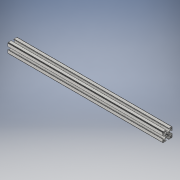
# Autodesk Inventor part: 30x30_extrude_horizontal_481mm
Saved by Autodesk Inventor 2016 (Build 200138000, 138)
## iProperties
Created: 2016-10-05
Part Number: 30x30_extrude_horizontal_481mm
Material: Generic
Document SubType Name: Modeling
Designer: gmmar
Density: 1 g/cm^3
Appearance: Default
Author: gmmar
Autodesk Inventor part; units mm, degrees
ref_plane "YZ Plane" through (0, 0, 0) normal (1, 0, 0) x (0, 1, 0)
ref_plane "XZ Plane" through (0, 0, 0) normal (0, 1, 0) x (-1, 0, 0)
ref_plane "XY Plane" through (0, 0, 0) normal (0, 0, 1) x (1, 0, 0)
sketch "Sketch1" plane through (0, 0, 0) normal (1, 0, 0) x (0, 1, 0)
  line L0 (12.7969, -8.25) -> (12.7969, -4)
  line L1 (-12.8031, 4) -> (-12.8031, 8.25)
  line L2 (-13.849, -12.8949) -> (-13.85, -12.85)
  line L3 (9.701, -12.8949) -> (9.7, -12.85)
  line L4 (-9.7, -10.7) -> (-9.701, -10.6551)
  line L5 (13.85, -10.7) -> (13.849, -10.6551)
  line L6 (9.701, 10.6551) -> (9.7, 10.7)
  line L7 (-13.849, 10.6551) -> (-13.85, 10.7)
  line L8 (13.85, 12.85) -> (13.849, 12.8949)
  line L9 (-9.7, 12.85) -> (-9.701, 12.8949)
  line L10 (-14.998, -13.0897) -> (-15, -13)
  line L11 (15, 13) -> (14.998, 13.0897)
  line L12 (9.704, -12.9396) -> (9.701, -12.8949)
  line L13 (-9.701, -10.6551) -> (-9.704, -10.6104)
  line L14 (9.704, 10.6104) -> (9.701, 10.6551)
  line L15 (-9.701, 12.8949) -> (-9.704, 12.9396)
  line L16 (-14.9919, -13.1793) -> (-14.998, -13.0897)
  line L17 (14.998, 13.0897) -> (14.9919, 13.1793)
  line L18 (-13.846, -12.9396) -> (-13.849, -12.8949)
  line L19 (13.849, -10.6551) -> (13.846, -10.6104)
  line L20 (-13.846, 10.6104) -> (-13.849, 10.6551)
  line L21 (13.849, 12.8949) -> (13.846, 12.9396)
  line L22 (13.846, -10.6104) -> (13.8409, -10.5658)
  line L23 (-13.8409, 10.5658) -> (-13.846, 10.6104)
  line L24 (-13.8409, -12.9842) -> (-13.846, -12.9396)
  line L25 (13.846, 12.9396) -> (13.8409, 12.9842)
  line L26 (-14.9819, -13.2685) -> (-14.9919, -13.1793)
  line L27 (14.9919, 13.1793) -> (14.9819, 13.2685)
  line L28 (-9.704, -10.6104) -> (-9.7091, -10.5658)
  line L29 (9.7091, 10.5658) -> (9.704, 10.6104)
  line L30 (9.7091, -12.9842) -> (9.704, -12.9396)
  line L31 (-9.704, 12.9396) -> (-9.7091, 12.9842)
  line L32 (-13.8339, -13.0286) -> (-13.8409, -12.9842)
  line L33 (9.7161, -13.0286) -> (9.7091, -12.9842)
  line L34 (13.8409, 12.9842) -> (13.8339, 13.0286)
  line L35 (-9.7091, 12.9842) -> (-9.7161, 13.0286)
  line L36 (-14.9679, -13.3571) -> (-14.9819, -13.2685)
  line L37 (14.9819, 13.2685) -> (14.9679, 13.3571)
  line L38 (-9.7091, -10.5658) -> (-9.7161, -10.5214)
  line L39 (13.8409, -10.5658) -> (13.8339, -10.5214)
  line L40 (9.7161, 10.5214) -> (9.7091, 10.5658)
  line L41 (-13.8339, 10.5214) -> (-13.8409, 10.5658)
  line L42 (-14.9499, -13.445) -> (-14.9679, -13.3571)
  line L43 (14.9679, 13.3571) -> (14.9499, 13.445)
  line L44 (-13.8249, -13.0725) -> (-13.8339, -13.0286)
  line L45 (9.7251, -13.0725) -> (9.7161, -13.0286)
  line L46 (-9.7161, -10.5214) -> (-9.7251, -10.4775)
  line L47 (13.8339, -10.5214) -> (13.8249, -10.4775)
  line L48 (9.7251, 10.4775) -> (9.7161, 10.5214)
  line L49 (-13.8249, 10.4775) -> (-13.8339, 10.5214)
  line L50 (13.8339, 13.0286) -> (13.8249, 13.0725)
  line L51 (-9.7161, 13.0286) -> (-9.7251, 13.0725)
  line L52 (-14.9279, -13.5321) -> (-14.9499, -13.445)
  line L53 (-9.7251, -10.4775) -> (-9.736, -10.434)
  line L54 (13.8249, -10.4775) -> (13.814, -10.434)
  line L55 (9.736, 10.434) -> (9.7251, 10.4775)
  line L56 (-13.814, 10.434) -> (-13.8249, 10.4775)
  line L57 (14.9499, 13.445) -> (14.9279, 13.5321)
  line L58 (-13.814, -13.116) -> (-13.8249, -13.0725)
  line L59 (9.736, -13.116) -> (9.7251, -13.0725)
  line L60 (13.8249, 13.0725) -> (13.814, 13.116)
  line L61 (-9.7251, 13.0725) -> (-9.736, 13.116)
  line L62 (-13.8011, -13.159) -> (-13.814, -13.116)
  line L63 (9.7489, -13.159) -> (9.736, -13.116)
  line L64 (13.814, 13.116) -> (13.8011, 13.159)
  line L65 (-9.736, 13.116) -> (-9.7489, 13.159)
  line L66 (-9.736, -10.434) -> (-9.7489, -10.391)
  line L67 (13.814, -10.434) -> (13.8011, -10.391)
  line L68 (9.7489, 10.391) -> (9.736, 10.434)
  line L69 (-13.8011, 10.391) -> (-13.814, 10.434)
  line L70 (-14.9021, -13.618) -> (-14.9279, -13.5321)
  line L71 (14.9279, 13.5321) -> (14.9021, 13.618)
  line L72 (-14.8725, -13.7027) -> (-14.9021, -13.618)
  line L73 (14.9021, 13.618) -> (14.8725, 13.7027)
  line L74 (-13.7862, -13.2014) -> (-13.8011, -13.159)
  line L75 (9.7638, -13.2014) -> (9.7489, -13.159)
  line L76 (-9.7489, -10.391) -> (-9.7638, -10.3486)
  line L77 (13.8011, -10.391) -> (13.7862, -10.3486)
  line L78 (9.7638, 10.3486) -> (9.7489, 10.391)
  line L79 (-13.7862, 10.3486) -> (-13.8011, 10.391)
  line L80 (13.8011, 13.159) -> (13.7862, 13.2014)
  line L81 (-9.7489, 13.159) -> (-9.7638, 13.2014)
  line L82 (-14.8391, -13.7861) -> (-14.8725, -13.7027)
  line L83 (14.8725, 13.7027) -> (14.8391, 13.7861)
  line L84 (9.7805, -13.243) -> (9.7638, -13.2014)
  line L85 (-9.7638, -10.3486) -> (-9.7805, -10.307)
  line L86 (9.7805, 10.307) -> (9.7638, 10.3486)
  line L87 (-9.7638, 13.2014) -> (-9.7805, 13.243)
  line L88 (-13.7695, -13.243) -> (-13.7862, -13.2014)
  line L89 (13.7862, -10.3486) -> (13.7695, -10.307)
  line L90 (-13.7695, 10.307) -> (-13.7862, 10.3486)
  line L91 (13.7862, 13.2014) -> (13.7695, 13.243)
  line L92 (-13.751, -13.2839) -> (-13.7695, -13.243)
  line L93 (13.7695, -10.307) -> (13.751, -10.2661)
  line L94 (-13.751, 10.2661) -> (-13.7695, 10.307)
  line L95 (13.7695, 13.243) -> (13.751, 13.2839)
  line L96 (9.799, -13.2839) -> (9.7805, -13.243)
  line L97 (-9.7805, -10.307) -> (-9.799, -10.2661)
  line L98 (9.799, 10.2661) -> (9.7805, 10.307)
  line L99 (-9.7805, 13.243) -> (-9.799, 13.2839)
  line L100 (-14.8019, -13.8678) -> (-14.8391, -13.7861)
  line L101 (14.8391, 13.7861) -> (14.8019, 13.8678)
  line L102 (-13.7306, -13.3239) -> (-13.751, -13.2839)
  line L103 (13.751, -10.2661) -> (13.7306, -10.2261)
  line L104 (-13.7306, 10.2261) -> (-13.751, 10.2661)
  line L105 (13.751, 13.2839) -> (13.7306, 13.3239)
  line L106 (-14.7612, -13.9477) -> (-14.8019, -13.8678)
  line L107 (14.8019, 13.8678) -> (14.7612, 13.9477)
  line L108 (9.8194, -13.3239) -> (9.799, -13.2839)
  line L109 (-9.799, -10.2661) -> (-9.8194, -10.2261)
  line L110 (9.8194, 10.2261) -> (9.799, 10.2661)
  line L111 (-9.799, 13.2839) -> (-9.8194, 13.3239)
  line L112 (-9.8194, -10.2261) -> (-9.8416, -10.1871)
  line L113 (9.8416, 10.1871) -> (9.8194, 10.2261)
  line L114 (9.8416, -13.3629) -> (9.8194, -13.3239)
  line L115 (-9.8194, 13.3239) -> (-9.8416, 13.3629)
  line L116 (-14.7169, -14.0258) -> (-14.7612, -13.9477)
  line L117 (14.7612, 13.9477) -> (14.7169, 14.0258)
  line L118 (13.7306, -10.2261) -> (13.7084, -10.1871)
  line L119 (-13.7084, 10.1871) -> (-13.7306, 10.2261)
  line L120 (-13.7084, -13.3629) -> (-13.7306, -13.3239)
  line L121 (13.7306, 13.3239) -> (13.7084, 13.3629)
  line L122 (6, -0.9196) -> (5.4782, 0)
  line L123 (-5.4782, 0) -> (-6, 0.9196)
  line L124 (-13.6846, -13.4009) -> (-13.7084, -13.3629)
  line L125 (13.7084, 13.3629) -> (13.6846, 13.4009)
  line L126 (13.7084, -10.1871) -> (13.6846, -10.1491)
  line L127 (-13.6846, 10.1491) -> (-13.7084, 10.1871)
  line L128 (-14.6691, -14.1018) -> (-14.7169, -14.0258)
  line L129 (14.7169, 14.0258) -> (14.6691, 14.1018)
  line L130 (9.8654, -13.4009) -> (9.8416, -13.3629)
  line L131 (-9.8416, 13.3629) -> (-9.8654, 13.4009)
  line L132 (-9.8416, -10.1871) -> (-9.8654, -10.1491)
  line L133 (9.8654, 10.1491) -> (9.8416, 10.1871)
  line L134 (-13.659, -13.4378) -> (-13.6846, -13.4009)
  line L135 (9.891, -13.4378) -> (9.8654, -13.4009)
  line L136 (-9.8654, -10.1491) -> (-9.891, -10.1122)
  line L137 (13.6846, -10.1491) -> (13.659, -10.1122)
  line L138 (9.891, 10.1122) -> (9.8654, 10.1491)
  line L139 (-13.659, 10.1122) -> (-13.6846, 10.1491)
  line L140 (13.6846, 13.4009) -> (13.659, 13.4378)
  line L141 (-9.8654, 13.4009) -> (-9.891, 13.4378)
  line L142 (-14.618, -14.1756) -> (-14.6691, -14.1018)
  line L143 (14.6691, 14.1018) -> (14.618, 14.1756)
  line L144 (-4.3624, -3.3495) -> (-4.5314, -3.1172)
  line L145 (4.5284, 3.125) -> (4.3639, 3.3512)
  line L146 (9.9182, -13.4735) -> (9.891, -13.4378)
  line L147 (-9.891, -10.1122) -> (-9.9182, -10.0765)
  line L148 (9.9182, 10.0765) -> (9.891, 10.1122)
  line L149 (-9.891, 13.4378) -> (-9.9182, 13.4735)
  line L150 (-14.5637, -14.247) -> (-14.618, -14.1756)
  line L151 (14.618, 14.1756) -> (14.5637, 14.247)
  line L152 (-13.6318, -13.4735) -> (-13.659, -13.4378)
  line L153 (13.659, -10.1122) -> (13.6318, -10.0765)
  line L154 (-13.6318, 10.0765) -> (-13.659, 10.1122)
  line L155 (13.659, 13.4378) -> (13.6318, 13.4735)
  line L156 (-4.1783, -3.57) -> (-4.3624, -3.3495)
  line L157 (4.3639, 3.3512) -> (4.1798, 3.5718)
  line L158 (-14.5061, -14.3159) -> (-14.5637, -14.247)
  line L159 (13.6318, -10.0765) -> (13.6031, -10.0421)
  line L160 (-13.6031, 10.0421) -> (-13.6318, 10.0765)
  line L161 (14.5637, 14.247) -> (14.5061, 14.3159)
  line L162 (-13.6031, -13.5079) -> (-13.6318, -13.4735)
  line L163 (13.6318, 13.4735) -> (13.6031, 13.5079)
  line L164 (-9.9182, -10.0765) -> (-9.9469, -10.0421)
  line L165 (9.9469, 10.0421) -> (9.9182, 10.0765)
  line L166 (9.9469, -13.5079) -> (9.9182, -13.4735)
  line L167 (-9.9182, 13.4735) -> (-9.9469, 13.5079)
  line L168 (4.5328, -3.1128) -> (3.2776, -1.6092)
  line L169 (-3.2762, 1.6197) -> (-4.5315, 3.1232)
  line L170 (-3.9845, -3.7821) -> (-4.1783, -3.57)
  line L171 (4.1798, 3.5718) -> (3.986, 3.7838)
  line L172 (-13.5728, -13.5411) -> (-13.6031, -13.5079)
  line L173 (9.9772, -13.5411) -> (9.9469, -13.5079)
  line L174 (-9.9469, -10.0421) -> (-9.9772, -10.0089)
  line L175 (13.6031, -10.0421) -> (13.5728, -10.0089)
  line L176 (9.9772, 10.0089) -> (9.9469, 10.0421)
  line L177 (-13.5728, 10.0089) -> (-13.6031, 10.0421)
  line L178 (13.6031, 13.5079) -> (13.5728, 13.5411)
  line L179 (-9.9469, 13.5079) -> (-9.9772, 13.5411)
  line L180 (-14.4456, -14.3821) -> (-14.5061, -14.3159)
  line L181 (14.5061, 14.3159) -> (14.4456, 14.3821)
  line L182 (10.0089, -13.5728) -> (9.9772, -13.5411)
  line L183 (-9.9772, 13.5411) -> (-10.0089, 13.5728)
  line L184 (-14.3821, -14.4456) -> (-14.4456, -14.3821)
  line L185 (-13.5411, -13.5728) -> (-13.5728, -13.5411)
  line L186 (8.25, -10.0531) -> (4.1969, -6)
  line L187 (-9.9772, -10.0089) -> (-10.0089, -9.9772)
  line L188 (10.0531, -8.25) -> (6, -4.1969)
  line L189 (-3.7814, -3.9852) -> (-3.9845, -3.7821)
  line L190 (3.986, 3.7838) -> (3.7828, 3.987)
  line L191 (-6, 4.1969) -> (-10.0531, 8.25)
  line L192 (-4.1969, 6) -> (-8.25, 10.0531)
  line L193 (10.0089, 9.9772) -> (9.9772, 10.0089)
  line L194 (13.5728, 13.5411) -> (13.5411, 13.5728)
  line L195 (14.4456, 14.3821) -> (14.3821, 14.4456)
  line L196 (13.5728, -10.0089) -> (13.5411, -9.9772)
  line L197 (-13.5411, 9.9772) -> (-13.5728, 10.0089)
  line L198 (-14.3159, -14.5061) -> (-14.3821, -14.4456)
  line L199 (14.3821, 14.4456) -> (14.3159, 14.5061)
  line L200 (-13.5079, -13.6031) -> (-13.5411, -13.5728)
  line L201 (10.0421, -13.6031) -> (10.0089, -13.5728)
  line L202 (-10.0089, -9.9772) -> (-10.0421, -9.9469)
  line L203 (13.5411, -9.9772) -> (13.5079, -9.9469)
  line L204 (10.0421, 9.9469) -> (10.0089, 9.9772)
  line L205 (-13.5079, 9.9469) -> (-13.5411, 9.9772)
  line L206 (13.5411, 13.5728) -> (13.5079, 13.6031)
  line L207 (-10.0089, 13.5728) -> (-10.0421, 13.6031)
  line L208 (-3.5693, -4.179) -> (-3.7814, -3.9852)
  line L209 (3.7828, 3.987) -> (3.5708, 4.1808)
  line L210 (3.1179, -4.5277) -> (1.6143, -3.2725)
  line L211 (-1.613, 3.283) -> (-3.1165, 4.5382)
  line L212 (13.5079, -9.9469) -> (13.4735, -9.9182)
  line L213 (-13.4735, 9.9182) -> (-13.5079, 9.9469)
  line L214 (-10.0421, -9.9469) -> (-10.0765, -9.9182)
  line L215 (10.0765, 9.9182) -> (10.0421, 9.9469)
  line L216 (-13.4735, -13.6318) -> (-13.5079, -13.6031)
  line L217 (13.5079, 13.6031) -> (13.4735, 13.6318)
  line L218 (-14.247, -14.5637) -> (-14.3159, -14.5061)
  line L219 (10.0765, -13.6318) -> (10.0421, -13.6031)
  line L220 (-10.0421, 13.6031) -> (-10.0765, 13.6318)
  line L221 (14.3159, 14.5061) -> (14.247, 14.5637)
  line L222 (-3.3488, -4.3632) -> (-3.5693, -4.179)
  line L223 (3.5708, 4.1808) -> (3.3502, 4.3649)
  line L224 (-13.4378, -13.659) -> (-13.4735, -13.6318)
  line L225 (10.1122, -13.659) -> (10.0765, -13.6318)
  line L226 (13.4735, 13.6318) -> (13.4378, 13.659)
  line L227 (-10.0765, 13.6318) -> (-10.1122, 13.659)
  line L228 (-14.1756, -14.618) -> (-14.247, -14.5637)
  line L229 (14.247, 14.5637) -> (14.1756, 14.618)
  line L230 (-10.0765, -9.9182) -> (-10.1122, -9.891)
  line L231 (13.4735, -9.9182) -> (13.4378, -9.891)
  line L232 (10.1122, 9.891) -> (10.0765, 9.9182)
  line L233 (-13.4378, 9.891) -> (-13.4735, 9.9182)
  line L234 (-3.1164, -4.5321) -> (-3.3488, -4.3632)
  line L235 (3.3502, 4.3649) -> (3.1179, 4.5338)
  line L236 (-14.1018, -14.6691) -> (-14.1756, -14.618)
  line L237 (14.1756, 14.618) -> (14.1018, 14.6691)
  line L238 (-13.4009, -13.6846) -> (-13.4378, -13.659)
  line L239 (10.1491, -13.6846) -> (10.1122, -13.659)
  line L240 (-10.1122, -9.891) -> (-10.1491, -9.8654)
  line L241 (13.4378, -9.891) -> (13.4009, -9.8654)
  line L242 (10.1491, 9.8654) -> (10.1122, 9.891)
  line L243 (-13.4009, 9.8654) -> (-13.4378, 9.891)
  line L244 (13.4378, 13.659) -> (13.4009, 13.6846)
  line L245 (-10.1122, 13.659) -> (-10.1491, 13.6846)
  line L246 (-10.1491, -9.8654) -> (-10.1871, -9.8416)
  line L247 (10.1871, 9.8416) -> (10.1491, 9.8654)
  line L248 (13.4009, -9.8654) -> (13.3629, -9.8416)
  line L249 (-13.3629, 9.8416) -> (-13.4009, 9.8654)
  line L250 (-14.0258, -14.7169) -> (-14.1018, -14.6691)
  line L251 (14.1018, 14.6691) -> (14.0258, 14.7169)
  line L252 (10.1871, -13.7084) -> (10.1491, -13.6846)
  line L253 (-10.1491, 13.6846) -> (-10.1871, 13.7084)
  line L254 (-13.3629, -13.7084) -> (-13.4009, -13.6846)
  line L255 (13.4009, 13.6846) -> (13.3629, 13.7084)
  line L256 (0.9196, -6) -> (0, -5.4782)
  line L257 (0, 5.4782) -> (-0.9196, 6)
  line L258 (-13.3239, -13.7306) -> (-13.3629, -13.7084)
  line L259 (13.3629, 13.7084) -> (13.3239, 13.7306)
  line L260 (10.2261, -13.7306) -> (10.1871, -13.7084)
  line L261 (-10.1871, 13.7084) -> (-10.2261, 13.7306)
  line L262 (-13.9477, -14.7612) -> (-14.0258, -14.7169)
  line L263 (14.0258, 14.7169) -> (13.9477, 14.7612)
  line L264 (13.3629, -9.8416) -> (13.3239, -9.8194)
  line L265 (-13.3239, 9.8194) -> (-13.3629, 9.8416)
  line L266 (-10.1871, -9.8416) -> (-10.2261, -9.8194)
  line L267 (10.2261, 9.8194) -> (10.1871, 9.8416)
  line L268 (-10.2261, -9.8194) -> (-10.2661, -9.799)
  line L269 (13.3239, -9.8194) -> (13.2839, -9.799)
  line L270 (10.2661, 9.799) -> (10.2261, 9.8194)
  line L271 (-13.2839, 9.799) -> (-13.3239, 9.8194)
  line L272 (-13.8678, -14.8019) -> (-13.9477, -14.7612)
  line L273 (13.9477, 14.7612) -> (13.8678, 14.8019)
  line L274 (-13.2839, -13.751) -> (-13.3239, -13.7306)
  line L275 (10.2661, -13.751) -> (10.2261, -13.7306)
  line L276 (13.3239, 13.7306) -> (13.2839, 13.751)
  line L277 (-10.2261, 13.7306) -> (-10.2661, 13.751)
  line L278 (-13.7861, -14.8391) -> (-13.8678, -14.8019)
  line L279 (13.8678, 14.8019) -> (13.7861, 14.8391)
  line L280 (-10.2661, -9.799) -> (-10.307, -9.7805)
  line L281 (13.2839, -9.799) -> (13.243, -9.7805)
  line L282 (10.307, 9.7805) -> (10.2661, 9.799)
  line L283 (-13.243, 9.7805) -> (-13.2839, 9.799)
  line L284 (-13.243, -13.7695) -> (-13.2839, -13.751)
  line L285 (10.307, -13.7695) -> (10.2661, -13.751)
  line L286 (13.2839, 13.751) -> (13.243, 13.7695)
  line L287 (-10.2661, 13.751) -> (-10.307, 13.7695)
  line L288 (-13.2014, -13.7862) -> (-13.243, -13.7695)
  line L289 (10.3486, -13.7862) -> (10.307, -13.7695)
  line L290 (13.243, 13.7695) -> (13.2014, 13.7862)
  line L291 (-10.307, 13.7695) -> (-10.3486, 13.7862)
  line L292 (-10.307, -9.7805) -> (-10.3486, -9.7638)
  line L293 (13.243, -9.7805) -> (13.2014, -9.7638)
  line L294 (10.3486, 9.7638) -> (10.307, 9.7805)
  line L295 (-13.2014, 9.7638) -> (-13.243, 9.7805)
  line L296 (-13.7027, -14.8725) -> (-13.7861, -14.8391)
  line L297 (13.7861, 14.8391) -> (13.7027, 14.8725)
  line L298 (-13.159, -13.8011) -> (-13.2014, -13.7862)
  line L299 (10.391, -13.8011) -> (10.3486, -13.7862)
  line L300 (-10.3486, -9.7638) -> (-10.391, -9.7489)
  line L301 (13.2014, -9.7638) -> (13.159, -9.7489)
  line L302 (10.391, 9.7489) -> (10.3486, 9.7638)
  line L303 (-13.159, 9.7489) -> (-13.2014, 9.7638)
  line L304 (13.2014, 13.7862) -> (13.159, 13.8011)
  line L305 (-10.3486, 13.7862) -> (-10.391, 13.8011)
  line L306 (-13.618, -14.9021) -> (-13.7027, -14.8725)
  line L307 (13.7027, 14.8725) -> (13.618, 14.9021)
  line L308 (-13.5321, -14.9279) -> (-13.618, -14.9021)
  line L309 (13.618, 14.9021) -> (13.5321, 14.9279)
  line L310 (10.434, -13.814) -> (10.391, -13.8011)
  line L311 (-10.391, -9.7489) -> (-10.434, -9.736)
  line L312 (10.434, 9.736) -> (10.391, 9.7489)
  line L313 (-10.391, 13.8011) -> (-10.434, 13.814)
  line L314 (-13.116, -13.814) -> (-13.159, -13.8011)
  line L315 (13.159, -9.7489) -> (13.116, -9.736)
  line L316 (-13.116, 9.736) -> (-13.159, 9.7489)
  line L317 (13.159, 13.8011) -> (13.116, 13.814)
  line L318 (-13.0725, -13.8249) -> (-13.116, -13.814)
  line L319 (13.116, -9.736) -> (13.0725, -9.7251)
  line L320 (-13.0725, 9.7251) -> (-13.116, 9.736)
  line L321 (13.116, 13.814) -> (13.0725, 13.8249)
  line L322 (-13.445, -14.9499) -> (-13.5321, -14.9279)
  line L323 (10.4775, -13.8249) -> (10.434, -13.814)
  line L324 (-10.434, -9.736) -> (-10.4775, -9.7251)
  line L325 (10.4775, 9.7251) -> (10.434, 9.736)
  line L326 (-10.434, 13.814) -> (-10.4775, 13.8249)
  line L327 (13.5321, 14.9279) -> (13.445, 14.9499)
  line L328 (-13.0286, -13.8339) -> (-13.0725, -13.8249)
  line L329 (10.5214, -13.8339) -> (10.4775, -13.8249)
  line L330 (-10.4775, -9.7251) -> (-10.5214, -9.7161)
  line L331 (13.0725, -9.7251) -> (13.0286, -9.7161)
  line L332 (10.5214, 9.7161) -> (10.4775, 9.7251)
  line L333 (-13.0286, 9.7161) -> (-13.0725, 9.7251)
  line L334 (13.0725, 13.8249) -> (13.0286, 13.8339)
  line L335 (-10.4775, 13.8249) -> (-10.5214, 13.8339)
  line L336 (-13.3571, -14.9679) -> (-13.445, -14.9499)
  line L337 (13.445, 14.9499) -> (13.3571, 14.9679)
  line L338 (10.5658, -13.8409) -> (10.5214, -13.8339)
  line L339 (-10.5214, -9.7161) -> (-10.5658, -9.7091)
  line L340 (10.5658, 9.7091) -> (10.5214, 9.7161)
  line L341 (-10.5214, 13.8339) -> (-10.5658, 13.8409)
  line L342 (-13.2685, -14.9819) -> (-13.3571, -14.9679)
  line L343 (13.3571, 14.9679) -> (13.2685, 14.9819)
  line L344 (-12.9842, -13.8409) -> (-13.0286, -13.8339)
  line L345 (13.0286, -9.7161) -> (12.9842, -9.7091)
  line L346 (-12.9842, 9.7091) -> (-13.0286, 9.7161)
  line L347 (13.0286, 13.8339) -> (12.9842, 13.8409)
  line L348 (12.9842, -9.7091) -> (12.9396, -9.704)
  line L349 (-12.9396, 9.704) -> (-12.9842, 9.7091)
  line L350 (-10.5658, -9.7091) -> (-10.6104, -9.704)
  line L351 (10.6104, 9.704) -> (10.5658, 9.7091)
  line L352 (-13.1793, -14.9919) -> (-13.2685, -14.9819)
  line L353 (13.2685, 14.9819) -> (13.1793, 14.9919)
  line L354 (-12.9396, -13.846) -> (-12.9842, -13.8409)
  line L355 (12.9842, 13.8409) -> (12.9396, 13.846)
  line L356 (10.6104, -13.846) -> (10.5658, -13.8409)
  line L357 (-10.5658, 13.8409) -> (-10.6104, 13.846)
  line L358 (-13.0897, -14.998) -> (-13.1793, -14.9919)
  line L359 (-12.8949, -13.849) -> (-12.9396, -13.846)
  line L360 (10.6551, -13.849) -> (10.6104, -13.846)
  line L361 (12.9396, 13.846) -> (12.8949, 13.849)
  line L362 (-10.6104, 13.846) -> (-10.6551, 13.849)
  line L363 (13.1793, 14.9919) -> (13.0897, 14.998)
  line L364 (-10.6104, -9.704) -> (-10.6551, -9.701)
  line L365 (12.9396, -9.704) -> (12.8949, -9.701)
  line L366 (10.6551, 9.701) -> (10.6104, 9.704)
  line L367 (-12.8949, 9.701) -> (-12.9396, 9.704)
  line L368 (-13, -15) -> (-13.0897, -14.998)
  line L369 (-12.85, -13.85) -> (-12.8949, -13.849)
  line L370 (10.7, -13.85) -> (10.6551, -13.849)
  line L371 (-10.6551, -9.701) -> (-10.7, -9.7)
  line L372 (12.8949, -9.701) -> (12.85, -9.7)
  line L373 (10.7, 9.7) -> (10.6551, 9.701)
  line L374 (-12.85, 9.7) -> (-12.8949, 9.701)
  line L375 (12.8949, 13.849) -> (12.85, 13.85)
  line L376 (-10.6551, 13.849) -> (-10.7, 13.85)
  line L377 (13.0897, 14.998) -> (13, 15)
  line L378 (8.25, -12.8031) -> (4, -12.8031)
  line L379 (-4, 12.8031) -> (-8.25, 12.8031)
  line L380 (-13, -15) -> (-4.5, -15)
  line L381 (4.5, -15) -> (13, -15)
  line L382 (-4.5, -14.5) -> (-4, -14.5)
  line L383 (4, -14.5) -> (4.5, -14.5)
  line L384 (-12.85, -13.85) -> (-10.7, -13.85)
  line L385 (10.7, -13.85) -> (12.85, -13.85)
  line L386 (-12.85, -9.7) -> (-10.7, -9.7)
  line L387 (10.7, -9.7) -> (12.85, -9.7)
  line L388 (-12.8031, -8.25) -> (-10.0531, -8.25)
  line L389 (10.0531, -8.25) -> (12.7969, -8.25)
  line L390 (-4.1969, -6) -> (-0.9196, -6)
  line L391 (0.9196, -6) -> (4.1969, -6)
  line L392 (-15, -4.5) -> (-14.5, -4.5)
  line L393 (14.5, -4.5) -> (15, -4.5)
  line L394 (-14.5, -4) -> (-12.8031, -4)
  line L395 (12.7969, -4) -> (14.5, -4)
  line L396 (12.7969, 4) -> (14.5, 4)
  line L397 (-14.5, 4) -> (-12.8031, 4)
  line L398 (14.5, 4.5) -> (15, 4.5)
  line L399 (-15, 4.5) -> (-14.5, 4.5)
  line L400 (0.9196, 6) -> (4.1969, 6)
  line L401 (-4.1969, 6) -> (-0.9196, 6)
  line L402 (10.0531, 8.25) -> (12.7969, 8.25)
  line L403 (-12.8031, 8.25) -> (-10.0531, 8.25)
  line L404 (10.7, 9.7) -> (12.85, 9.7)
  line L405 (-12.85, 9.7) -> (-10.7, 9.7)
  line L406 (10.7, 13.85) -> (12.85, 13.85)
  line L407 (-12.85, 13.85) -> (-10.7, 13.85)
  line L408 (4, 14.5) -> (4.5, 14.5)
  line L409 (-4.5, 14.5) -> (-4, 14.5)
  line L410 (4.5, 15) -> (13, 15)
  line L411 (-13, 15) -> (-4.5, 15)
  line L412 (-8.25, -12.8031) -> (-4, -12.8031)
  line L413 (4, 12.7969) -> (8.25, 12.7969)
  line L414 (13, -15) -> (13.0897, -14.998)
  line L415 (-10.7, -13.85) -> (-10.6551, -13.849)
  line L416 (12.85, -13.85) -> (12.8949, -13.849)
  line L417 (-12.8949, -9.701) -> (-12.85, -9.7)
  line L418 (10.6551, -9.701) -> (10.7, -9.7)
  line L419 (12.85, 9.7) -> (12.8949, 9.701)
  line L420 (-10.7, 9.7) -> (-10.6551, 9.701)
  line L421 (10.6551, 13.849) -> (10.7, 13.85)
  line L422 (-12.8949, 13.849) -> (-12.85, 13.85)
  line L423 (-13.0897, 14.998) -> (-13, 15)
  line L424 (-12.9396, -9.704) -> (-12.8949, -9.701)
  line L425 (10.6104, -9.704) -> (10.6551, -9.701)
  line L426 (12.8949, 9.701) -> (12.9396, 9.704)
  line L427 (-10.6551, 9.701) -> (-10.6104, 9.704)
  line L428 (13.0897, -14.998) -> (13.1793, -14.9919)
  line L429 (-10.6551, -13.849) -> (-10.6104, -13.846)
  line L430 (12.8949, -13.849) -> (12.9396, -13.846)
  line L431 (10.6104, 13.846) -> (10.6551, 13.849)
  line L432 (-12.9396, 13.846) -> (-12.8949, 13.849)
  line L433 (-13.1793, 14.9919) -> (-13.0897, 14.998)
  line L434 (-10.6104, -13.846) -> (-10.5658, -13.8409)
  line L435 (10.5658, 13.8409) -> (10.6104, 13.846)
  line L436 (12.9396, -13.846) -> (12.9842, -13.8409)
  line L437 (-12.9842, 13.8409) -> (-12.9396, 13.846)
  line L438 (13.1793, -14.9919) -> (13.2685, -14.9819)
  line L439 (-13.2685, 14.9819) -> (-13.1793, 14.9919)
  line L440 (10.5658, -9.7091) -> (10.6104, -9.704)
  line L441 (-10.6104, 9.704) -> (-10.5658, 9.7091)
  line L442 (-12.9842, -9.7091) -> (-12.9396, -9.704)
  line L443 (12.9396, 9.704) -> (12.9842, 9.7091)
  line L444 (12.9842, -13.8409) -> (13.0286, -13.8339)
  line L445 (-13.0286, -9.7161) -> (-12.9842, -9.7091)
  line L446 (12.9842, 9.7091) -> (13.0286, 9.7161)
  line L447 (-13.0286, 13.8339) -> (-12.9842, 13.8409)
  line L448 (13.2685, -14.9819) -> (13.3571, -14.9679)
  line L449 (-13.3571, 14.9679) -> (-13.2685, 14.9819)
  line L450 (-10.5658, -13.8409) -> (-10.5214, -13.8339)
  line L451 (10.5214, -9.7161) -> (10.5658, -9.7091)
  line L452 (-10.5658, 9.7091) -> (-10.5214, 9.7161)
  line L453 (10.5214, 13.8339) -> (10.5658, 13.8409)
  line L454 (13.3571, -14.9679) -> (13.445, -14.9499)
  line L455 (-13.445, 14.9499) -> (-13.3571, 14.9679)
  line L456 (-10.5214, -13.8339) -> (-10.4775, -13.8249)
  line L457 (13.0286, -13.8339) -> (13.0725, -13.8249)
  line L458 (-13.0725, -9.7251) -> (-13.0286, -9.7161)
  line L459 (10.4775, -9.7251) -> (10.5214, -9.7161)
  line L460 (13.0286, 9.7161) -> (13.0725, 9.7251)
  line L461 (-10.5214, 9.7161) -> (-10.4775, 9.7251)
  line L462 (10.4775, 13.8249) -> (10.5214, 13.8339)
  line L463 (-13.0725, 13.8249) -> (-13.0286, 13.8339)
  line L464 (13.445, -14.9499) -> (13.5321, -14.9279)
  line L465 (-10.4775, -13.8249) -> (-10.434, -13.814)
  line L466 (10.434, -9.736) -> (10.4775, -9.7251)
  line L467 (-10.4775, 9.7251) -> (-10.434, 9.736)
  line L468 (10.434, 13.814) -> (10.4775, 13.8249)
  line L469 (-13.5321, 14.9279) -> (-13.445, 14.9499)
  line L470 (13.0725, -13.8249) -> (13.116, -13.814)
  line L471 (-13.116, -9.736) -> (-13.0725, -9.7251)
  line L472 (13.0725, 9.7251) -> (13.116, 9.736)
  line L473 (-13.116, 13.814) -> (-13.0725, 13.8249)
  line L474 (13.116, -13.814) -> (13.159, -13.8011)
  line L475 (-13.159, -9.7489) -> (-13.116, -9.736)
  line L476 (13.116, 9.736) -> (13.159, 9.7489)
  line L477 (-13.159, 13.8011) -> (-13.116, 13.814)
  line L478 (-10.434, -13.814) -> (-10.391, -13.8011)
  line L479 (10.391, -9.7489) -> (10.434, -9.736)
  line L480 (-10.434, 9.736) -> (-10.391, 9.7489)
  line L481 (10.391, 13.8011) -> (10.434, 13.814)
  line L482 (13.5321, -14.9279) -> (13.618, -14.9021)
  line L483 (-13.618, 14.9021) -> (-13.5321, 14.9279)
  line L484 (13.618, -14.9021) -> (13.7027, -14.8725)
  line L485 (-13.7027, 14.8725) -> (-13.618, 14.9021)
  line L486 (-10.391, -13.8011) -> (-10.3486, -13.7862)
  line L487 (13.159, -13.8011) -> (13.2014, -13.7862)
  line L488 (-13.2014, -9.7638) -> (-13.159, -9.7489)
  line L489 (10.3486, -9.7638) -> (10.391, -9.7489)
  line L490 (13.159, 9.7489) -> (13.2014, 9.7638)
  line L491 (-10.391, 9.7489) -> (-10.3486, 9.7638)
  line L492 (10.3486, 13.7862) -> (10.391, 13.8011)
  line L493 (-13.2014, 13.7862) -> (-13.159, 13.8011)
  line L494 (13.7027, -14.8725) -> (13.7861, -14.8391)
  line L495 (-13.7861, 14.8391) -> (-13.7027, 14.8725)
  line L496 (-13.243, -9.7805) -> (-13.2014, -9.7638)
  line L497 (10.307, -9.7805) -> (10.3486, -9.7638)
  line L498 (13.2014, 9.7638) -> (13.243, 9.7805)
  line L499 (-10.3486, 9.7638) -> (-10.307, 9.7805)
  line L500 (-10.3486, -13.7862) -> (-10.307, -13.7695)
  line L501 (13.2014, -13.7862) -> (13.243, -13.7695)
  line L502 (10.307, 13.7695) -> (10.3486, 13.7862)
  line L503 (-13.243, 13.7695) -> (-13.2014, 13.7862)
  line L504 (-10.307, -13.7695) -> (-10.2661, -13.751)
  line L505 (13.243, -13.7695) -> (13.2839, -13.751)
  line L506 (10.2661, 13.751) -> (10.307, 13.7695)
  line L507 (-13.2839, 13.751) -> (-13.243, 13.7695)
  line L508 (-13.2839, -9.799) -> (-13.243, -9.7805)
  line L509 (10.2661, -9.799) -> (10.307, -9.7805)
  line L510 (13.243, 9.7805) -> (13.2839, 9.799)
  line L511 (-10.307, 9.7805) -> (-10.2661, 9.799)
  line L512 (13.7861, -14.8391) -> (13.8678, -14.8019)
  line L513 (-13.8678, 14.8019) -> (-13.7861, 14.8391)
  line L514 (-10.2661, -13.751) -> (-10.2261, -13.7306)
  line L515 (13.2839, -13.751) -> (13.3239, -13.7306)
  line L516 (10.2261, 13.7306) -> (10.2661, 13.751)
  line L517 (-13.3239, 13.7306) -> (-13.2839, 13.751)
  line L518 (13.8678, -14.8019) -> (13.9477, -14.7612)
  line L519 (-13.9477, 14.7612) -> (-13.8678, 14.8019)
  line L520 (-13.3239, -9.8194) -> (-13.2839, -9.799)
  line L521 (10.2261, -9.8194) -> (10.2661, -9.799)
  line L522 (13.2839, 9.799) -> (13.3239, 9.8194)
  line L523 (-10.2661, 9.799) -> (-10.2261, 9.8194)
  line L524 (10.1871, -9.8416) -> (10.2261, -9.8194)
  line L525 (-10.2261, 9.8194) -> (-10.1871, 9.8416)
  line L526 (-13.3629, -9.8416) -> (-13.3239, -9.8194)
  line L527 (13.3239, 9.8194) -> (13.3629, 9.8416)
  line L528 (13.9477, -14.7612) -> (14.0258, -14.7169)
  line L529 (-14.0258, 14.7169) -> (-13.9477, 14.7612)
  line L530 (-10.2261, -13.7306) -> (-10.1871, -13.7084)
  line L531 (10.1871, 13.7084) -> (10.2261, 13.7306)
  line L532 (13.3239, -13.7306) -> (13.3629, -13.7084)
  line L533 (-13.3629, 13.7084) -> (-13.3239, 13.7306)
  line L534 (-0.9196, -6) -> (0, -5.4782)
  line L535 (0, 5.4782) -> (0.9196, 6)
  line L536 (13.3629, -13.7084) -> (13.4009, -13.6846)
  line L537 (-13.4009, 13.6846) -> (-13.3629, 13.7084)
  line L538 (-10.1871, -13.7084) -> (-10.1491, -13.6846)
  line L539 (10.1491, 13.6846) -> (10.1871, 13.7084)
  line L540 (14.0258, -14.7169) -> (14.1018, -14.6691)
  line L541 (-14.1018, 14.6691) -> (-14.0258, 14.7169)
  line L542 (-13.4009, -9.8654) -> (-13.3629, -9.8416)
  line L543 (13.3629, 9.8416) -> (13.4009, 9.8654)
  line L544 (10.1491, -9.8654) -> (10.1871, -9.8416)
  line L545 (-10.1871, 9.8416) -> (-10.1491, 9.8654)
  line L546 (-10.1491, -13.6846) -> (-10.1122, -13.659)
  line L547 (13.4009, -13.6846) -> (13.4378, -13.659)
  line L548 (-13.4378, -9.891) -> (-13.4009, -9.8654)
  line L549 (10.1122, -9.891) -> (10.1491, -9.8654)
  line L550 (13.4009, 9.8654) -> (13.4378, 9.891)
  line L551 (-10.1491, 9.8654) -> (-10.1122, 9.891)
  line L552 (10.1122, 13.659) -> (10.1491, 13.6846)
  line L553 (-13.4378, 13.659) -> (-13.4009, 13.6846)
  line L554 (14.1018, -14.6691) -> (14.1756, -14.618)
  line L555 (-14.1756, 14.618) -> (-14.1018, 14.6691)
  line L556 (3.1179, -4.5277) -> (3.3502, -4.3588)
  line L557 (-3.3489, 4.3692) -> (-3.1165, 4.5382)
  line L558 (-13.4735, -9.9182) -> (-13.4378, -9.891)
  line L559 (10.0765, -9.9182) -> (10.1122, -9.891)
  line L560 (13.4378, 9.891) -> (13.4735, 9.9182)
  line L561 (-10.1122, 9.891) -> (-10.0765, 9.9182)
  line L562 (14.1756, -14.618) -> (14.247, -14.5637)
  line L563 (-14.247, 14.5637) -> (-14.1756, 14.618)
  line L564 (-10.1122, -13.659) -> (-10.0765, -13.6318)
  line L565 (13.4378, -13.659) -> (13.4735, -13.6318)
  line L566 (10.0765, 13.6318) -> (10.1122, 13.659)
  line L567 (-13.4735, 13.6318) -> (-13.4378, 13.659)
  line L568 (3.3502, -4.3588) -> (3.5707, -4.1747)
  line L569 (-3.5694, 4.1851) -> (-3.3489, 4.3692)
  line L570 (14.247, -14.5637) -> (14.3159, -14.5061)
  line L571 (-10.0765, -13.6318) -> (-10.0421, -13.6031)
  line L572 (10.0421, 13.6031) -> (10.0765, 13.6318)
  line L573 (-14.3159, 14.5061) -> (-14.247, 14.5637)
  line L574 (13.4735, -13.6318) -> (13.5079, -13.6031)
  line L575 (-13.5079, 13.6031) -> (-13.4735, 13.6318)
  line L576 (10.0421, -9.9469) -> (10.0765, -9.9182)
  line L577 (-10.0765, 9.9182) -> (-10.0421, 9.9469)
  line L578 (-13.5079, -9.9469) -> (-13.4735, -9.9182)
  line L579 (13.4735, 9.9182) -> (13.5079, 9.9469)
  line L580 (-3.1164, -4.5321) -> (-1.6129, -3.2769)
  line L581 (1.6144, 3.2786) -> (3.1179, 4.5338)
  line L582 (3.5707, -4.1747) -> (3.7828, -3.9808)
  line L583 (-3.7814, 3.9913) -> (-3.5694, 4.1851)
  line L584 (-10.0421, -13.6031) -> (-10.0089, -13.5728)
  line L585 (13.5079, -13.6031) -> (13.5411, -13.5728)
  line L586 (-13.5411, -9.9772) -> (-13.5079, -9.9469)
  line L587 (10.0089, -9.9772) -> (10.0421, -9.9469)
  line L588 (13.5079, 9.9469) -> (13.5411, 9.9772)
  line L589 (-10.0421, 9.9469) -> (-10.0089, 9.9772)
  line L590 (10.0089, 13.5728) -> (10.0421, 13.6031)
  line L591 (-13.5411, 13.5728) -> (-13.5079, 13.6031)
  line L592 (14.3159, -14.5061) -> (14.3821, -14.4456)
  line L593 (-14.3821, 14.4456) -> (-14.3159, 14.5061)
  line L594 (-13.5728, -10.0089) -> (-13.5411, -9.9772)
  line L595 (13.5411, 9.9772) -> (13.5728, 10.0089)
  line L596 (14.3821, -14.4456) -> (14.4456, -14.3821)
  line L597 (13.5411, -13.5728) -> (13.5728, -13.5411)
  line L598 (-8.25, -10.0531) -> (-4.1969, -6)
  line L599 (9.9772, -10.0089) -> (10.0089, -9.9772)
  line L600 (-10.0531, -8.25) -> (-6, -4.1969)
  line L601 (3.7828, -3.9808) -> (3.9859, -3.7777)
  line L602 (-3.9846, 3.7882) -> (-3.7814, 3.9913)
  line L603 (6, 4.1969) -> (10.0531, 8.25)
  line L604 (4.1969, 6) -> (8.25, 10.0531)
  line L605 (-10.0089, 9.9772) -> (-9.9772, 10.0089)
  line L606 (-13.5728, 13.5411) -> (-13.5411, 13.5728)
  line L607 (-14.4456, 14.3821) -> (-14.3821, 14.4456)
  line L608 (-10.0089, -13.5728) -> (-9.9772, -13.5411)
  line L609 (9.9772, 13.5411) -> (10.0089, 13.5728)
  line L610 (14.4456, -14.3821) -> (14.5061, -14.3159)
  line L611 (-14.5061, 14.3159) -> (-14.4456, 14.3821)
  line L612 (-9.9772, -13.5411) -> (-9.9469, -13.5079)
  line L613 (13.5728, -13.5411) -> (13.6031, -13.5079)
  line L614 (-13.6031, -10.0421) -> (-13.5728, -10.0089)
  line L615 (9.9469, -10.0421) -> (9.9772, -10.0089)
  line L616 (13.5728, 10.0089) -> (13.6031, 10.0421)
  line L617 (-9.9772, 10.0089) -> (-9.9469, 10.0421)
  line L618 (9.9469, 13.5079) -> (9.9772, 13.5411)
  line L619 (-13.6031, 13.5079) -> (-13.5728, 13.5411)
  line L620 (3.9859, -3.7777) -> (4.1797, -3.5657)
  line L621 (-4.1784, 3.5761) -> (-3.9846, 3.7882)
  line L622 (-4.5314, -3.1172) -> (-3.2761, -1.6136)
  line L623 (3.2741, 1.6226) -> (4.5284, 3.125)
  line L624 (-9.9469, -13.5079) -> (-9.9182, -13.4735)
  line L625 (9.9182, 13.4735) -> (9.9469, 13.5079)
  line L626 (9.9182, -10.0765) -> (9.9469, -10.0421)
  line L627 (-9.9469, 10.0421) -> (-9.9182, 10.0765)
  line L628 (13.6031, -13.5079) -> (13.6318, -13.4735)
  line L629 (-13.6318, 13.4735) -> (-13.6031, 13.5079)
  line L630 (14.5061, -14.3159) -> (14.5637, -14.247)
  line L631 (-13.6318, -10.0765) -> (-13.6031, -10.0421)
  line L632 (13.6031, 10.0421) -> (13.6318, 10.0765)
  line L633 (-14.5637, 14.247) -> (-14.5061, 14.3159)
  line L634 (4.1797, -3.5657) -> (4.3639, -3.3451)
  line L635 (-4.3625, 3.3556) -> (-4.1784, 3.5761)
  line L636 (13.6318, -13.4735) -> (13.659, -13.4378)
  line L637 (-13.659, -10.1122) -> (-13.6318, -10.0765)
  line L638 (13.6318, 10.0765) -> (13.659, 10.1122)
  line L639 (-13.659, 13.4378) -> (-13.6318, 13.4735)
  line L640 (14.5637, -14.247) -> (14.618, -14.1756)
  line L641 (-14.618, 14.1756) -> (-14.5637, 14.247)
  line L642 (-9.9182, -13.4735) -> (-9.891, -13.4378)
  line L643 (9.891, -10.1122) -> (9.9182, -10.0765)
  line L644 (-9.9182, 10.0765) -> (-9.891, 10.1122)
  line L645 (9.891, 13.4378) -> (9.9182, 13.4735)
  line L646 (4.3639, -3.3451) -> (4.5328, -3.1128)
  line L647 (-4.5315, 3.1232) -> (-4.3625, 3.3556)
  line L648 (14.618, -14.1756) -> (14.6691, -14.1018)
  line L649 (-14.6691, 14.1018) -> (-14.618, 14.1756)
  line L650 (-9.891, -13.4378) -> (-9.8654, -13.4009)
  line L651 (13.659, -13.4378) -> (13.6846, -13.4009)
  line L652 (-13.6846, -10.1491) -> (-13.659, -10.1122)
  line L653 (9.8654, -10.1491) -> (9.891, -10.1122)
  line L654 (13.659, 10.1122) -> (13.6846, 10.1491)
  line L655 (-9.891, 10.1122) -> (-9.8654, 10.1491)
  line L656 (9.8654, 13.4009) -> (9.891, 13.4378)
  line L657 (-13.6846, 13.4009) -> (-13.659, 13.4378)
  line L658 (9.8416, -10.1871) -> (9.8654, -10.1491)
  line L659 (-9.8654, 10.1491) -> (-9.8416, 10.1871)
  line L660 (-9.8654, -13.4009) -> (-9.8416, -13.3629)
  line L661 (9.8416, 13.3629) -> (9.8654, 13.4009)
  line L662 (14.6691, -14.1018) -> (14.7169, -14.0258)
  line L663 (-14.7169, 14.0258) -> (-14.6691, 14.1018)
  line L664 (-13.7084, -10.1871) -> (-13.6846, -10.1491)
  line L665 (13.6846, 10.1491) -> (13.7084, 10.1871)
  line L666 (13.6846, -13.4009) -> (13.7084, -13.3629)
  line L667 (-13.7084, 13.3629) -> (-13.6846, 13.4009)
  line L668 (-6, -0.9196) -> (-5.4782, 0)
  line L669 (5.4782, 0) -> (6, 0.9196)
  line L670 (13.7084, -13.3629) -> (13.7306, -13.3239)
  line L671 (-13.7306, 13.3239) -> (-13.7084, 13.3629)
  line L672 (-13.7306, -10.2261) -> (-13.7084, -10.1871)
  line L673 (13.7084, 10.1871) -> (13.7306, 10.2261)
  line L674 (14.7169, -14.0258) -> (14.7612, -13.9477)
  line L675 (-14.7612, 13.9477) -> (-14.7169, 14.0258)
  line L676 (-9.8416, -13.3629) -> (-9.8194, -13.3239)
  line L677 (9.8194, 13.3239) -> (9.8416, 13.3629)
  line L678 (9.8194, -10.2261) -> (9.8416, -10.1871)
  line L679 (-9.8416, 10.1871) -> (-9.8194, 10.2261)
  line L680 (-9.8194, -13.3239) -> (-9.799, -13.2839)
  line L681 (9.799, -10.2661) -> (9.8194, -10.2261)
  line L682 (-9.8194, 10.2261) -> (-9.799, 10.2661)
  line L683 (9.799, 13.2839) -> (9.8194, 13.3239)
  line L684 (14.7612, -13.9477) -> (14.8019, -13.8678)
  line L685 (-14.8019, 13.8678) -> (-14.7612, 13.9477)
  line L686 (13.7306, -13.3239) -> (13.751, -13.2839)
  line L687 (-13.751, -10.2661) -> (-13.7306, -10.2261)
  line L688 (13.7306, 10.2261) -> (13.751, 10.2661)
  line L689 (-13.751, 13.2839) -> (-13.7306, 13.3239)
  line L690 (14.8019, -13.8678) -> (14.8391, -13.7861)
  line L691 (-14.8391, 13.7861) -> (-14.8019, 13.8678)
  line L692 (-9.799, -13.2839) -> (-9.7805, -13.243)
  line L693 (9.7805, -10.307) -> (9.799, -10.2661)
  line L694 (-9.799, 10.2661) -> (-9.7805, 10.307)
  line L695 (9.7805, 13.243) -> (9.799, 13.2839)
  line L696 (13.751, -13.2839) -> (13.7695, -13.243)
  line L697 (-13.7695, -10.307) -> (-13.751, -10.2661)
  line L698 (13.751, 10.2661) -> (13.7695, 10.307)
  line L699 (-13.7695, 13.243) -> (-13.751, 13.2839)
  line L700 (13.7695, -13.243) -> (13.7862, -13.2014)
  line L701 (-13.7862, -10.3486) -> (-13.7695, -10.307)
  line L702 (13.7695, 10.307) -> (13.7862, 10.3486)
  line L703 (-13.7862, 13.2014) -> (-13.7695, 13.243)
  line L704 (-9.7805, -13.243) -> (-9.7638, -13.2014)
  line L705 (9.7638, -10.3486) -> (9.7805, -10.307)
  line L706 (-9.7805, 10.307) -> (-9.7638, 10.3486)
  line L707 (9.7638, 13.2014) -> (9.7805, 13.243)
  line L708 (14.8391, -13.7861) -> (14.8725, -13.7027)
  line L709 (-14.8725, 13.7027) -> (-14.8391, 13.7861)
  line L710 (-9.7638, -13.2014) -> (-9.7489, -13.159)
  line L711 (13.7862, -13.2014) -> (13.8011, -13.159)
  line L712 (-13.8011, -10.391) -> (-13.7862, -10.3486)
  line L713 (9.7489, -10.391) -> (9.7638, -10.3486)
  line L714 (13.7862, 10.3486) -> (13.8011, 10.391)
  line L715 (-9.7638, 10.3486) -> (-9.7489, 10.391)
  line L716 (9.7489, 13.159) -> (9.7638, 13.2014)
  line L717 (-13.8011, 13.159) -> (-13.7862, 13.2014)
  line L718 (14.8725, -13.7027) -> (14.9021, -13.618)
  line L719 (-14.9021, 13.618) -> (-14.8725, 13.7027)
  line L720 (14.9021, -13.618) -> (14.9279, -13.5321)
  line L721 (-14.9279, 13.5321) -> (-14.9021, 13.618)
  line L722 (-13.814, -10.434) -> (-13.8011, -10.391)
  line L723 (9.736, -10.434) -> (9.7489, -10.391)
  line L724 (13.8011, 10.391) -> (13.814, 10.434)
  line L725 (-9.7489, 10.391) -> (-9.736, 10.434)
  line L726 (-9.7489, -13.159) -> (-9.736, -13.116)
  line L727 (13.8011, -13.159) -> (13.814, -13.116)
  line L728 (9.736, 13.116) -> (9.7489, 13.159)
  line L729 (-13.814, 13.116) -> (-13.8011, 13.159)
  line L730 (-9.736, -13.116) -> (-9.7251, -13.0725)
  line L731 (13.814, -13.116) -> (13.8249, -13.0725)
  line L732 (9.7251, 13.0725) -> (9.736, 13.116)
  line L733 (-13.8249, 13.0725) -> (-13.814, 13.116)
  line L734 (14.9279, -13.5321) -> (14.9499, -13.445)
  line L735 (-13.8249, -10.4775) -> (-13.814, -10.434)
  line L736 (9.7251, -10.4775) -> (9.736, -10.434)
  line L737 (13.814, 10.434) -> (13.8249, 10.4775)
  line L738 (-9.736, 10.434) -> (-9.7251, 10.4775)
  line L739 (-14.9499, 13.445) -> (-14.9279, 13.5321)
  line L740 (-9.7251, -13.0725) -> (-9.7161, -13.0286)
  line L741 (13.8249, -13.0725) -> (13.8339, -13.0286)
  line L742 (-13.8339, -10.5214) -> (-13.8249, -10.4775)
  line L743 (9.7161, -10.5214) -> (9.7251, -10.4775)
  line L744 (13.8249, 10.4775) -> (13.8339, 10.5214)
  line L745 (-9.7251, 10.4775) -> (-9.7161, 10.5214)
  line L746 (9.7161, 13.0286) -> (9.7251, 13.0725)
  line L747 (-13.8339, 13.0286) -> (-13.8249, 13.0725)
  line L748 (14.9499, -13.445) -> (14.9679, -13.3571)
  line L749 (-14.9679, 13.3571) -> (-14.9499, 13.445)
  line L750 (-13.8409, -10.5658) -> (-13.8339, -10.5214)
  line L751 (9.7091, -10.5658) -> (9.7161, -10.5214)
  line L752 (13.8339, 10.5214) -> (13.8409, 10.5658)
  line L753 (-9.7161, 10.5214) -> (-9.7091, 10.5658)
  line L754 (14.9679, -13.3571) -> (14.9819, -13.2685)
  line L755 (-14.9819, 13.2685) -> (-14.9679, 13.3571)
  line L756 (-9.7161, -13.0286) -> (-9.7091, -12.9842)
  line L757 (13.8339, -13.0286) -> (13.8409, -12.9842)
  line L758 (9.7091, 12.9842) -> (9.7161, 13.0286)
  line L759 (-13.8409, 12.9842) -> (-13.8339, 13.0286)
  line L760 (-9.7091, -12.9842) -> (-9.704, -12.9396)
  line L761 (9.704, 12.9396) -> (9.7091, 12.9842)
  line L762 (9.704, -10.6104) -> (9.7091, -10.5658)
  line L763 (-9.7091, 10.5658) -> (-9.704, 10.6104)
  line L764 (14.9819, -13.2685) -> (14.9919, -13.1793)
  line L765 (-14.9919, 13.1793) -> (-14.9819, 13.2685)
  line L766 (13.8409, -12.9842) -> (13.846, -12.9396)
  line L767 (-13.846, 12.9396) -> (-13.8409, 12.9842)
  line L768 (-13.846, -10.6104) -> (-13.8409, -10.5658)
  line L769 (13.8409, 10.5658) -> (13.846, 10.6104)
  line L770 (13.846, -12.9396) -> (13.849, -12.8949)
  line L771 (-13.849, -10.6551) -> (-13.846, -10.6104)
  line L772 (13.846, 10.6104) -> (13.849, 10.6551)
  line L773 (-13.849, 12.8949) -> (-13.846, 12.9396)
  line L774 (14.9919, -13.1793) -> (14.998, -13.0897)
  line L775 (-14.998, 13.0897) -> (-14.9919, 13.1793)
  line L776 (-9.704, -12.9396) -> (-9.701, -12.8949)
  line L777 (9.701, -10.6551) -> (9.704, -10.6104)
  line L778 (-9.704, 10.6104) -> (-9.701, 10.6551)
  line L779 (9.701, 12.8949) -> (9.704, 12.9396)
  line L780 (14.998, -13.0897) -> (15, -13)
  line L781 (-15, 13) -> (-14.998, 13.0897)
  line L782 (-9.701, -12.8949) -> (-9.7, -12.85)
  line L783 (13.849, -12.8949) -> (13.85, -12.85)
  line L784 (-13.85, -10.7) -> (-13.849, -10.6551)
  line L785 (9.7, -10.7) -> (9.701, -10.6551)
  line L786 (13.849, 10.6551) -> (13.85, 10.7)
  line L787 (-9.701, 10.6551) -> (-9.7, 10.7)
  line L788 (9.7, 12.85) -> (9.701, 12.8949)
  line L789 (-13.85, 12.85) -> (-13.849, 12.8949)
  line L790 (-12.8031, -8.25) -> (-12.8031, -4)
  line L791 (12.7969, 4) -> (12.7969, 8.25)
  line L792 (-15, 4.5) -> (-15, 13)
  line L793 (-15, -13) -> (-15, -4.5)
  line L794 (-14.5, 4) -> (-14.5, 4.5)
  line L795 (-14.5, -4.5) -> (-14.5, -4)
  line L796 (-13.85, -12.85) -> (-13.85, -10.7)
  line L797 (-13.85, 10.7) -> (-13.85, 12.85)
  line L798 (-9.7, -12.85) -> (-9.7, -10.7)
  line L799 (-9.7, 10.7) -> (-9.7, 12.85)
  line L800 (-8.25, 10.0531) -> (-8.25, 12.8031)
  line L801 (-8.25, -12.8031) -> (-8.25, -10.0531)
  line L802 (-6, 0.9196) -> (-6, 4.1969)
  line L803 (-6, -4.1969) -> (-6, -0.9196)
  line L804 (-4.5, 14.5) -> (-4.5, 15)
  line L805 (-4.5, -15) -> (-4.5, -14.5)
  line L806 (-4, 12.8031) -> (-4, 14.5)
  line L807 (-4, -14.5) -> (-4, -12.8031)
  line L808 (4, 12.7969) -> (4, 14.5)
  line L809 (4, -14.5) -> (4, -12.8031)
  line L810 (4.5, 14.5) -> (4.5, 15)
  line L811 (4.5, -15) -> (4.5, -14.5)
  line L812 (6, 0.9196) -> (6, 4.1969)
  line L813 (6, -4.1969) -> (6, -0.9196)
  line L814 (8.25, 10.0531) -> (8.25, 12.7969)
  line L815 (8.25, -12.8031) -> (8.25, -10.0531)
  line L816 (9.7, -12.85) -> (9.7, -10.7)
  line L817 (9.7, 10.7) -> (9.7, 12.85)
  line L818 (13.85, -12.85) -> (13.85, -10.7)
  line L819 (13.85, 10.7) -> (13.85, 12.85)
  line L820 (14.5, 4) -> (14.5, 4.5)
  line L821 (14.5, -4.5) -> (14.5, -4)
  line L822 (15, 4.5) -> (15, 13)
  line L823 (15, -13) -> (15, -4.5)
  arc A0 (-3.2762, 1.6197) -> (-3.2761, -1.6136) centre (-0.0037, 0.0031) ccw
  arc A1 (-1.6129, -3.2769) -> (1.6143, -3.2725) centre (-0.0037, 0.0031) ccw
  arc A2 (3.2776, -1.6092) -> (3.2741, 1.6226) centre (-0.0037, 0.0031) ccw
  arc A3 (1.6144, 3.2786) -> (-1.613, 3.283) centre (-0.0037, 0.0031) ccw
  point P0 (0, 0)
  constraints: 1648 end point, 708 parallel, 40 collinear, 8 point on circle, 4 centre point, 3 concentric, 1 horizontal, 1 vertical
extrude "Extrusion1" add sketch "Sketch1" along normal blind 481
body "Solid1"
